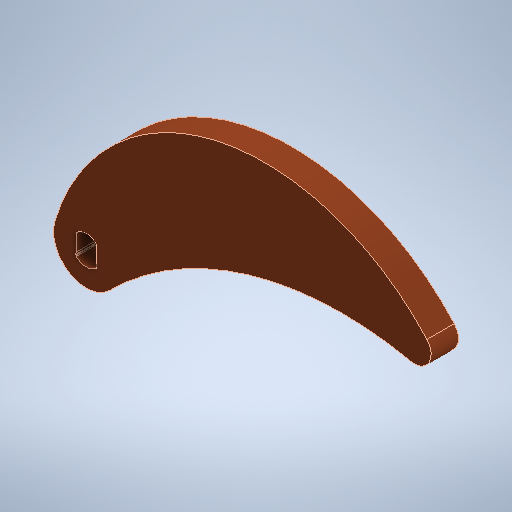
# Autodesk Inventor part: Shooting Arm
Saved by Autodesk Inventor 2025.4 (Build 294407000, 407)
## iProperties
Created: 2026-04-07
Part Number: Shooting Arm
Material: Generic
Document SubType Name: Sheet Metal
Designer: lenovo
Density: 1 g/cm^3
Sheet Metal Rule: Default_mm
Appearance: Default(1)
Author: lenovo
Autodesk Inventor part; units mm, degrees
ref_plane "YZ Plane" through (0, 0, 0) normal (1, 0, 0) x (0, 1, 0)
ref_plane "XZ Plane" through (0, 0, 0) normal (0, 1, 0) x (-1, 0, 0)
ref_plane "XY Plane" through (0, 0, 0) normal (0, 0, 1) x (1, 0, 0)
sketch "Sketch1" plane through (0, 0, 0) normal (0, 0, 1) x (1, 0, 0)
  line L0 (0, 2.65) -> (0, -2.65)
  line L1 (-1.85, 0) -> (1.85, 0)
  line L2 (1.85, 1.8974) -> (1.85, -1.8974)
  arc A0 (1.85, 1.8974) -> (-1.85, 1.8974) centre (0, 0) ccw
  line L3 (-1.85, 1.8974) -> (-1.85, -1.8974)
  arc A1 (-1.85, -1.8974) -> (1.85, -1.8974) centre (0, 0) ccw
  arc A2 (-5.7447, 1.7317) -> (4.2498, -4.2355) centre (0, 0) ccw
  arc A3 (62.2254, 17.0118) -> (-5.7447, 1.7317) centre (32.5532, -9.8127) ccw
  arc A4 (59.3689, 12.0671) -> (4.2498, -4.2355) centre (46.7476, -46.5904) ccw
  arc A5 (59.3689, 12.0671) -> (62.2254, 17.0118) centre (60, 15) ccw
  circle A6 centre (0, 0) radius 1.6
  circle A7 centre (0, 0) radius 2.5
  arc A8 (2.492, 0.2) -> (1.5354, 0.45) centre (1.85, -0.3014) ccw
  arc A9 (1.5354, -0.45) -> (2.492, -0.2) centre (1.85, 0.3014) ccw
  arc A10 (1.6207, 1.9035) -> (0.7675, 1.4039) centre (1.5212, 1.095) ccw
  arc A11 (1.4039, 0.7675) -> (1.9035, 1.6207) centre (1.095, 1.5212) ccw
  arc A12 (-0.2, 2.492) -> (-0.45, 1.5354) centre (0.3014, 1.85) ccw
  arc A13 (0.45, 1.5354) -> (0.2, 2.492) centre (-0.3014, 1.85) ccw
  arc A14 (-1.9035, 1.6207) -> (-1.4039, 0.7675) centre (-1.095, 1.5212) ccw
  arc A15 (-0.7675, 1.4039) -> (-1.6207, 1.9035) centre (-1.5212, 1.095) ccw
  arc A16 (-2.492, -0.2) -> (-1.5354, -0.45) centre (-1.85, 0.3014) ccw
  arc A17 (-1.5354, 0.45) -> (-2.492, 0.2) centre (-1.85, -0.3014) ccw
  arc A18 (-1.6207, -1.9035) -> (-0.7675, -1.4039) centre (-1.5212, -1.095) ccw
  arc A19 (-1.4039, -0.7675) -> (-1.9035, -1.6207) centre (-1.095, -1.5212) ccw
  arc A20 (0.2, -2.492) -> (0.45, -1.5354) centre (-0.3014, -1.85) ccw
  arc A21 (-0.45, -1.5354) -> (-0.2, -2.492) centre (0.3014, -1.85) ccw
  arc A22 (1.9035, -1.6207) -> (1.4039, -0.7675) centre (1.095, -1.5212) ccw
  arc A23 (0.7675, -1.4039) -> (1.6207, -1.9035) centre (1.5212, -1.095) ccw
  line L4 (0, 2.65) -> (0, -2.65)
  arc A24 (1.85, 1.8974) -> (-1.85, 1.8974) centre (0, 0) ccw
  line L5 (-1.85, 0) -> (1.85, 0)
  line L6 (-1.85, 1.8974) -> (-1.85, -1.8974)
  arc A25 (-1.85, -1.8974) -> (1.85, -1.8974) centre (0, 0) ccw
  line L7 (1.85, 1.8974) -> (1.85, -1.8974)
  point P0 (1.85, 0)
  point P1 (-1.85, 1.6815)
  point P2 (-1.6207, 1.9035)
  point P3 (-0.45, 1.5354)
  point P4 (-0.2, 2.492)
  point P5 (0.2, 2.492)
  point P6 (0.7675, 1.4039)
  point P7 (1.9035, 1.6207)
  point P8 (2.492, -0.2)
  point P9 (1.5354, -0.45)
  point P10 (1.4039, -0.7675)
  point P11 (1.6207, -1.9035)
  point P12 (0.45, -1.5354)
  point P13 (0.2, -2.492)
  point P14 (-0.2, -2.492)
  point P15 (-0.7675, -1.4039)
  point P16 (-1.6207, -1.9035)
  point P17 (-1.9035, -1.6207)
  point P18 (-1.4039, -0.7675)
  point P19 (-1.5354, -0.45)
  point P20 (-2.492, 0.2)
  point P21 (-1.4039, 0.7675)
  point P22 (-1.85, 1.2154)
  point P23 (1.85, -1.2154)
  point P24 (1.85, -1.6815)
  point P25 (-1.85, -1.6815)
  point P26 (-1.85, -1.2154)
  dimension "d12" = 3.2
  dimension "d13" = 5
  dimension "d2" = 2.65
  dimension "d3" = 3.7
  dimension "d5" = 6
  dimension "d6" = 40
  dimension "d7" = 3
  dimension "d8" = 60
  dimension "d9" = 60
  dimension "d10" = 15
  dimension "d14" = 0.4
  dimension "d15" = 0.9
  dimension "d18" = 360
  dimension "d20" = 2.65
  dimension "d21" = 3.7
  measures "d2" radius of A0
  measures "d3" diameter of L2 L0
  measures "d5" radius of A2
  measures "d6" radius of A3
  measures "d7" radius of A5
  measures "d8" radius of A4
  measures "d9" horizontal distance of A5.centre point (0, 0)
  measures "d10" vertical distance of A5.centre point (0, 0)
  measures "d14" diameter of A8.start L1
  measures "d15" distance of A9.start A8.end
  measures "d20" radius of A24
  measures "d21" diameter of L7 L4
extrude "Plate1" add sketch "Sketch1" along normal mid plane 5 contours A7 A11 L2 | L3 A14 A7 | A11 A7 A8 L2 | L3 A17 A7 A14 | A8 A7 A9 L2 | L3 A16 A7 A17 | A16 L3 A19 A7 | A9 A7 A22 L2 | A3 A5 A4 A2
equation "\"d11\" = Thickness"
equation "\"BendRadius\" = Thickness"
equation "\"BendReliefWidth\" = Thickness"
equation "\"BendReliefDepth\" = 0.5 * Thickness"
equation "\"TransitionRadius\" = BendRadius"
equation "\"JacobiRadiusSize\" = BendRadius"
equation "\"GapSize\" = Thickness"
equation "\"Thickness\" = 5"
body "Solid1"
